Autodesk Fusion 360 part; units mm, degrees
(part 19 of 24)
  arc A6027 (67.5837, 18.8834) -> (67.2903, 18.7619) centre (67.437, 18.8226) ccw
  line L2242 (72.517, 13.6779) -> (72.517, 12.446)
  arc A6028 (74.5092, 15.1708) -> (74.6307, 14.8774) centre (74.57, 15.0241) ccw
  arc A6029 (72.6757, 12.446) -> (72.3582, 12.446) centre (72.517, 12.446) ccw
  line L2243 (78.673, 15.2859) -> (74.5249, 11.1379)
  arc A6030 (73.5901, 11.9357) -> (73.9076, 11.9357) centre (73.7489, 11.9357) ccw
  arc A6031 (75.5723, 15.8051) -> (75.5723, 15.4877) centre (75.5723, 15.6464) ccw
  arc A6032 (72.3583, 11.2141) -> (72.6758, 11.2141) centre (72.517, 11.2141) ccw
  arc A6033 (72.517, 11.3728) -> (72.517, 11.0554) centre (72.517, 11.2141) ccw
  line L2244 (74.5249, 11.1379) -> (72.1601, 11.1379)
  line L2245 (73.7489, 12.9563) -> (73.0273, 13.6779)
  line L2246 (75.2188, 15.2929) -> (75.5723, 15.6464)
  arc A6034 (72.517, 13.8366) -> (72.517, 13.5191) centre (72.517, 13.6779) ccw
  arc A6035 (73.7489, 12.2872) -> (73.7489, 12.6047) centre (73.7489, 12.446) ccw
  arc A6036 (72.517, 11.0553) -> (72.517, 11.3728) centre (72.517, 11.2141) ccw
  arc A6037 (73.9076, 12.9563) -> (73.5901, 12.9563) centre (73.7489, 12.9563) ccw
  line L2247 (72.517, 12.446) -> (72.517, 11.2141)
  arc A6038 (78.5607, 15.3982) -> (78.7852, 15.1737) centre (78.673, 15.286) ccw
  arc A6039 (72.1961, 11.3264) -> (71.9716, 11.1018) centre (72.0838, 11.2141) ccw
  line L2248 (73.0273, 13.6779) -> (72.517, 13.6779)
  arc A6040 (79.2149, 15.4997) -> (79.0934, 15.7931) centre (79.1542, 15.6464) ccw
  arc A6041 (73.8612, 11.8235) -> (73.6366, 12.048) centre (73.7489, 11.9358) ccw
  arc A6042 (72.1601, 11.2966) -> (72.1601, 10.9791) centre (72.1601, 11.1379) ccw
  line L2249 (75.5723, 15.6464) -> (79.1542, 15.6464)
  line L2250 (79.1542, 15.6464) -> (78.9481, 15.561)
  arc A6043 (75.1065, 15.4051) -> (75.331, 15.1806) centre (75.2188, 15.2929) ccw
  arc A6044 (79.1542, 15.4877) -> (79.1542, 15.8051) centre (79.1542, 15.6464) ccw
  line L2251 (78.9481, 15.561) -> (78.673, 15.2859)
  arc A6045 (74.5699, 14.8654) -> (74.5699, 15.1829) centre (74.5699, 15.0242) ccw
  arc A6046 (72.3583, 12.446) -> (72.6758, 12.446) centre (72.517, 12.446) ccw
  line L2252 (72.517, 11.2141) -> (73.0273, 11.2141)
  arc A6047 (73.1395, 13.7902) -> (72.915, 13.5656) centre (73.0272, 13.6779) ccw
  arc A6048 (74.5249, 10.9791) -> (74.5249, 11.2966) centre (74.5249, 11.1379) ccw
  arc A6049 (73.8677, 15.1829) -> (73.8677, 14.8654) centre (73.8677, 15.0242) ccw
  arc A6050 (73.9076, 12.446) -> (73.5901, 12.446) centre (73.7489, 12.446) ccw
  arc A6051 (78.8873, 15.7077) -> (79.0088, 15.4144) centre (78.948, 15.5611) ccw
  line L2253 (72.0839, 11.2141) -> (72.517, 11.2141)
  arc A6052 (72.0478, 11.0256) -> (72.2723, 11.2502) centre (72.16, 11.1379) ccw
  arc A6053 (72.517, 12.2872) -> (72.517, 12.6047) centre (72.517, 12.446) ccw
  arc A6054 (74.4127, 11.2502) -> (74.6372, 11.0256) centre (74.525, 11.1379) ccw
  arc A6055 (73.0273, 13.5191) -> (73.0273, 13.8366) centre (73.0273, 13.6779) ccw
  arc A6056 (72.6758, 12.446) -> (72.3583, 12.446) centre (72.517, 12.446) ccw
  arc A6057 (73.6366, 12.844) -> (73.8612, 13.0685) centre (73.7489, 12.9562) ccw
  arc A6058 (72.3582, 11.2141) -> (72.6757, 11.2141) centre (72.517, 11.2141) ccw
  arc A6059 (72.517, 12.6047) -> (72.517, 12.2872) centre (72.517, 12.446) ccw
  arc A6060 (72.3582, 12.446) -> (72.6757, 12.446) centre (72.517, 12.446) ccw
  arc A6061 (73.0273, 11.0554) -> (73.0273, 11.3728) centre (73.0273, 11.2141) ccw
  arc A6062 (78.7852, 15.1737) -> (78.5607, 15.3982) centre (78.673, 15.2859) ccw
  line L2254 (74.5699, 15.0241) -> (75.2188, 15.2929)
  arc A6063 (79.0603, 15.4488) -> (78.8358, 15.6733) centre (78.9481, 15.561) ccw
  line L2255 (73.7489, 11.9357) -> (73.7489, 12.446)
  line L2256 (72.517, 12.446) -> (73.7489, 12.446)
  arc A6064 (72.6757, 12.446) -> (72.3582, 12.446) centre (72.517, 12.446) ccw
  line L2257 (68.4989, 14.799) -> (68.1395, 14.9479)
  arc A6065 (71.1264, 12.0129) -> (71.4438, 12.0129) centre (71.2851, 12.0129) ccw
  arc A6066 (46.6957, 21.6967) -> (46.4024, 21.5752) centre (46.5491, 21.636) ccw
  line L2258 (72.517, 12.446) -> (72.517, 13.6779)
  arc A6067 (46.8566, 21.2765) -> (46.5391, 21.2765) centre (46.6979, 21.2765) ccw
  arc A6068 (72.517, 12.6048) -> (72.517, 12.2873) centre (72.517, 12.4461) ccw
  line L2259 (68.774, 14.5239) -> (68.4989, 14.799)
  arc A6069 (72.517, 12.6047) -> (72.517, 12.2872) centre (72.517, 12.446) ccw
  arc A6070 (68.6153, 14.5239) -> (68.9328, 14.5239) centre (68.7741, 14.5239) ccw
  arc A6071 (68.6618, 14.4117) -> (68.8863, 14.6362) centre (68.774, 14.524) ccw
  arc A6072 (72.915, 11.3264) -> (73.1395, 11.1018) centre (73.0272, 11.2141) ccw
  arc A6073 (46.8102, 18.2973) -> (46.5856, 18.0728) centre (46.6979, 18.185) ccw
  arc A6074 (46.5512, 21.2158) -> (46.8446, 21.3373) centre (46.6979, 21.2765) ccw
  line L2260 (46.6979, 21.2765) -> (46.549, 21.6359)
  line L2261 (72.0067, 13.6779) -> (71.2851, 12.9563)
  line L2262 (73.0273, 11.2141) -> (73.7489, 11.9357)
  arc A6075 (49.9351, 15.1066) -> (49.9351, 14.7891) centre (49.9351, 14.9479) ccw
  arc A6076 (68.8863, 14.6362) -> (68.6618, 14.4117) centre (68.7741, 14.5239) ccw
  arc A6077 (68.4382, 14.6524) -> (68.5597, 14.9457) centre (68.499, 14.7991) ccw
  line L2263 (49.9351, 14.9479) -> (46.6979, 18.1851)
  arc A6078 (72.3583, 12.446) -> (72.6758, 12.446) centre (72.517, 12.446) ccw
  arc A6079 (72.6757, 13.6779) -> (72.3582, 13.6779) centre (72.517, 13.6779) ccw
  arc A6080 (73.7489, 12.2873) -> (73.7489, 12.6048) centre (73.7489, 12.4461) ccw
  line L2264 (71.2851, 12.9563) -> (71.2851, 12.446)
  line L2265 (71.2851, 12.0129) -> (68.774, 14.5239)
  arc A6081 (72.6758, 12.446) -> (72.3583, 12.446) centre (72.517, 12.446) ccw
  line L2266 (73.7489, 12.446) -> (72.517, 12.446)
  line L2267 (72.1601, 11.1379) -> (72.0839, 11.2141)
  arc A6082 (72.0839, 11.3728) -> (72.0839, 11.0554) centre (72.0839, 11.2141) ccw
  arc A6083 (46.5391, 18.1851) -> (46.8566, 18.1851) centre (46.6979, 18.1851) ccw
  arc A6084 (72.517, 12.2873) -> (72.517, 12.6048) centre (72.517, 12.4461) ccw
  line L2268 (46.6979, 18.1851) -> (46.6979, 21.2765)
  arc A6085 (71.1728, 11.9006) -> (71.3974, 12.1251) centre (71.2851, 12.0129) ccw
  line L2269 (71.2851, 12.446) -> (71.2851, 12.0129)
  arc A6086 (72.3582, 12.446) -> (72.6757, 12.446) centre (72.517, 12.446) ccw
  arc A6087 (37.5797, 23.0188) -> (37.5797, 22.7012) centre (37.5797, 22.86) ccw
  arc A6088 (72.517, 13.5191) -> (72.517, 13.8366) centre (72.517, 13.6779) ccw
  arc A6089 (44.69, 23.6538) -> (44.69, 23.3362) centre (44.69, 23.495) ccw
  arc A6090 (36.0803, 22.7012) -> (36.0803, 23.0188) centre (36.0803, 22.86) ccw
  arc A6091 (29.21, 23.6538) -> (29.21, 23.3362) centre (29.21, 23.495) ccw
  arc A6092 (71.2851, 12.6047) -> (71.2851, 12.2872) centre (71.2851, 12.446) ccw
  arc A6093 (56.8579, 23.0188) -> (56.8579, 22.7012) centre (56.8579, 22.86) ccw
  line L2270 (71.2851, 12.446) -> (72.517, 12.446)
  arc A6094 (68.6112, 14.9113) -> (68.3867, 14.6868) centre (68.499, 14.799) ccw
  arc A6095 (72.517, 12.2872) -> (72.517, 12.6047) centre (72.517, 12.446) ccw
  arc A6096 (41.924, 23.3362) -> (41.924, 23.6538) centre (41.924, 23.495) ccw
  arc A6097 (49.8228, 14.8356) -> (50.0473, 15.0602) centre (49.9351, 14.9479) ccw
  arc A6098 (71.4438, 12.9563) -> (71.1264, 12.9563) centre (71.2851, 12.9563) ccw
  arc A6099 (32.4997, 23.0188) -> (32.4997, 22.7012) centre (32.4997, 22.86) ccw
  arc A6100 (47.5103, 22.7012) -> (47.5103, 23.0188) centre (47.5103, 22.86) ccw
  arc A6101 (68.2003, 15.0946) -> (68.0788, 14.8012) centre (68.1395, 14.9479) ccw
  arc A6102 (25.1591, 23.3362) -> (25.1591, 23.6538) centre (25.1591, 23.495) ccw
  arc A6103 (38.3409, 23.6538) -> (38.3409, 23.3362) centre (38.3409, 23.495) ccw
  arc A6104 (46.7491, 23.3362) -> (46.7491, 23.6538) centre (46.7491, 23.495) ccw
  line L2271 (72.517, 13.6779) -> (72.0067, 13.6779)
  arc A6105 (72.6758, 13.6779) -> (72.3583, 13.6779) centre (72.517, 13.6779) ccw
  arc A6106 (49.0097, 23.0188) -> (49.0097, 22.7012) centre (49.0097, 22.86) ccw
  line L2272 (72.517, 12.446) -> (71.2851, 12.446)
  arc A6107 (6.2857, 22.7012) -> (6.2857, 23.0188) centre (6.2857, 22.86) ccw
  arc A6108 (69.342, 22.7012) -> (69.342, 23.0188) centre (69.342, 22.86) ccw
  arc A6109 (68.1395, 14.7891) -> (68.1395, 15.1066) centre (68.1395, 14.9479) ccw
  arc A6110 (29.21, 23.3362) -> (29.21, 23.6538) centre (29.21, 23.495) ccw
  arc A6111 (72.0067, 13.8366) -> (72.0067, 13.5191) centre (72.0067, 13.6779) ccw
  arc A6112 (72.119, 13.5656) -> (71.8945, 13.7902) centre (72.0068, 13.6779) ccw
  arc A6113 (71.1264, 12.446) -> (71.4438, 12.446) centre (71.2851, 12.446) ccw
  arc A6114 (71.1728, 13.0685) -> (71.3974, 12.844) centre (71.2851, 12.9563) ccw
  arc A6115 (71.4438, 12.446) -> (71.1264, 12.446) centre (71.2851, 12.446) ccw
  arc A6116 (71.2851, 12.6048) -> (71.2851, 12.2873) centre (71.2851, 12.4461) ccw
  line L2273 (46.549, 21.6359) -> (46.2739, 21.911)
  line L2274 (12.3063, 33.5781) -> (12.5596, 32.9666)
  line L2275 (68.1395, 14.9479) -> (49.9351, 14.9479)
  arc A6117 (72.517, 12.2873) -> (72.517, 12.6048) centre (72.517, 12.4461) ccw
  arc A6118 (0.7747, 23.6538) -> (0.7747, 23.3362) centre (0.7747, 23.495) ccw
  arc A6119 (68.9328, 14.5239) -> (68.6153, 14.5239) centre (68.7741, 14.5239) ccw
  arc A6120 (7.62, 23.0188) -> (7.62, 22.7012) centre (7.62, 22.86) ccw
  arc A6121 (79.8488, 22.7012) -> (79.8488, 23.0188) centre (79.8488, 22.86) ccw
  arc A6122 (71.628, 24.2888) -> (71.628, 23.9713) centre (71.628, 24.1301) ccw
  arc A6123 (54.9021, 23.3362) -> (54.9021, 23.6538) centre (54.9021, 23.495) ccw
  arc A6124 (54.5068, 23.6538) -> (54.5068, 23.3362) centre (54.5068, 23.495) ccw
  arc A6125 (84.2253, 22.7012) -> (84.2253, 23.0188) centre (84.2253, 22.86) ccw
  arc A6126 (53.34, 23.3362) -> (53.34, 23.6538) centre (53.34, 23.495) ccw
  arc A6127 (71.628, 23.0188) -> (71.628, 22.7012) centre (71.628, 22.86) ccw
  arc A6128 (45.325, 23.0188) -> (45.325, 22.7012) centre (45.325, 22.86) ccw
  arc A6129 (25.9203, 22.7012) -> (25.9203, 23.0188) centre (25.9203, 22.86) ccw
  arc A6130 (33.5403, 22.7012) -> (33.5403, 23.0188) centre (33.5403, 22.86) ccw
  arc A6131 (42.559, 22.7012) -> (42.559, 23.0188) centre (42.559, 22.86) ccw
  arc A6132 (75.0912, 23.0188) -> (75.0912, 22.7012) centre (75.0912, 22.86) ccw
  arc A6133 (73.3464, 22.7012) -> (73.3464, 23.0188) centre (73.3464, 22.86) ccw
  arc A6134 (83.5279, 23.0188) -> (83.5279, 22.7012) centre (83.5279, 22.86) ccw
  arc A6135 (83.298, 22.3838) -> (83.298, 22.0663) centre (83.298, 22.2251) ccw
  arc A6136 (53.34, 23.6538) -> (53.34, 23.3362) centre (53.34, 23.495) ccw
  arc A6137 (0.7747, 23.0188) -> (0.7747, 22.7012) centre (0.7747, 22.86) ccw
  arc A6138 (27.4197, 23.0188) -> (27.4197, 22.7012) centre (27.4197, 22.86) ccw
  arc A6139 (54.9021, 22.7012) -> (54.9021, 23.0188) centre (54.9021, 22.86) ccw
  arc A6140 (7.62, 22.7012) -> (7.62, 23.0188) centre (7.62, 22.86) ccw
  arc A6141 (71.628, 22.3838) -> (71.628, 22.0663) centre (71.628, 22.2251) ccw
  arc A6142 (8.9543, 23.0188) -> (8.9543, 22.7012) centre (8.9543, 22.86) ccw
  arc A6143 (31.0003, 22.7012) -> (31.0003, 23.0188) centre (31.0003, 22.86) ccw
  arc A6144 (35.0397, 23.0188) -> (35.0397, 22.7012) centre (35.0397, 22.86) ccw
  arc A6145 (51.5497, 23.0188) -> (51.5497, 22.7012) centre (51.5497, 22.86) ccw
  arc A6146 (50.0503, 22.7012) -> (50.0503, 23.0188) centre (50.0503, 22.86) ccw
  arc A6147 (84.2253, 22.0663) -> (84.2253, 22.3838) centre (84.2253, 22.2251) ccw
  arc A6148 (44.972, 24.6062) -> (44.972, 24.9238) centre (44.972, 24.765) ccw
  arc A6149 (81.5721, 23.3362) -> (81.5721, 23.6538) centre (81.5721, 23.495) ccw
  arc A6150 (46.4947, 23.9713) -> (46.4947, 24.2888) centre (46.4947, 24.1301) ccw
  arc A6151 (29.21, 24.9238) -> (29.21, 24.6062) centre (29.21, 24.765) ccw
  arc A6152 (54.9021, 24.6062) -> (54.9021, 24.9238) centre (54.9021, 24.765) ccw
  arc A6153 (59.8864, 24.9238) -> (59.8864, 24.6062) centre (59.8864, 24.765) ccw
  arc A6154 (72.39, 24.6062) -> (72.39, 24.9238) centre (72.39, 24.765) ccw
  arc A6155 (56.8579, 23.6538) -> (56.8579, 23.3362) centre (56.8579, 23.495) ccw
  arc A6156 (24.9047, 23.9713) -> (24.9047, 24.2888) centre (24.9047, 24.1301) ccw
  arc A6157 (56.9536, 24.6062) -> (56.9536, 24.9238) centre (56.9536, 24.765) ccw
  arc A6158 (84.2253, 23.9713) -> (84.2253, 24.2888) centre (84.2253, 24.1301) ccw
  arc A6159 (40.816, 24.6062) -> (40.816, 24.9238) centre (40.816, 24.765) ccw
  arc A6160 (68.58, 24.6062) -> (68.58, 24.9238) centre (68.58, 24.765) ccw
  arc A6161 (53.34, 24.2888) -> (53.34, 23.9713) centre (53.34, 24.1301) ccw
  arc A6162 (44.055, 24.2888) -> (44.055, 23.9713) centre (44.055, 24.1301) ccw
  arc A6163 (43.42, 24.9238) -> (43.42, 24.6062) centre (43.42, 24.765) ccw
  arc A6164 (53.34, 24.9238) -> (53.34, 24.6062) centre (53.34, 24.765) ccw
  arc A6165 (69.342, 23.9713) -> (69.342, 24.2888) centre (69.342, 24.1301) ccw
  arc A6166 (41.289, 23.9713) -> (41.289, 24.2888) centre (41.289, 24.1301) ccw
  arc A6167 (57.5886, 23.9713) -> (57.5886, 24.2888) centre (57.5886, 24.1301) ccw
  arc A6168 (54.9021, 23.9713) -> (54.9021, 24.2888) centre (54.9021, 24.1301) ccw
  arc A6169 (38.5953, 24.9238) -> (38.5953, 24.6062) centre (38.5953, 24.765) ccw
  arc A6170 (54.8513, 24.9238) -> (54.8513, 24.6062) centre (54.8513, 24.765) ccw
  arc A6171 (72.39, 24.9238) -> (72.39, 24.6062) centre (72.39, 24.765) ccw
  arc A6172 (53.34, 24.6062) -> (53.34, 24.9238) centre (53.34, 24.765) ccw
  arc A6173 (67.4728, 24.6062) -> (67.4728, 24.9238) centre (67.4728, 24.765) ccw
  arc A6174 (68.58, 24.9238) -> (68.58, 24.6062) centre (68.58, 24.765) ccw
  arc A6175 (54.8178, 24.2888) -> (54.8178, 23.9713) centre (54.8178, 24.1301) ccw
  arc A6176 (71.628, 23.6538) -> (71.628, 23.3362) centre (71.628, 23.495) ccw
  arc A6177 (0.7747, 24.2888) -> (0.7747, 23.9713) centre (0.7747, 24.1301) ccw
  arc A6178 (83.5279, 24.2888) -> (83.5279, 23.9713) centre (83.5279, 24.1301) ccw
  arc A6179 (54.9021, 25.2413) -> (54.9021, 25.5588) centre (54.9021, 25.4001) ccw
  arc A6180 (59.2514, 24.2888) -> (59.2514, 23.9713) centre (59.2514, 24.1301) ccw
  arc A6181 (83.5279, 23.6538) -> (83.5279, 23.3362) centre (83.5279, 23.495) ccw
  arc A6182 (43.1637, 25.5588) -> (43.1637, 25.2413) centre (43.1637, 25.4001) ccw
  arc A6183 (0.7747, 24.9238) -> (0.7747, 24.6062) centre (0.7747, 24.765) ccw
  arc A6184 (81.5721, 23.9713) -> (81.5721, 24.2888) centre (81.5721, 24.1301) ccw
  arc A6185 (56.8579, 24.2888) -> (56.8579, 23.9713) centre (56.8579, 24.1301) ccw
  arc A6186 (84.0359, 25.5588) -> (84.0359, 25.2413) centre (84.0359, 25.4001) ccw
  arc A6187 (59.8864, 26.1938) -> (59.8864, 25.8762) centre (59.8864, 26.035) ccw
  arc A6188 (29.21, 24.2888) -> (29.21, 23.9713) centre (29.21, 24.1301) ccw
  arc A6189 (84.2253, 23.3362) -> (84.2253, 23.6538) centre (84.2253, 23.495) ccw
  arc A6190 (56.8579, 24.9238) -> (56.8579, 24.6062) centre (56.8579, 24.765) ccw
  arc A6191 (68.58, 25.8762) -> (68.58, 26.1938) centre (68.58, 26.035) ccw
  arc A6192 (15.4854, 24.6062) -> (15.4854, 24.9238) centre (15.4854, 24.765) ccw
  arc A6193 (73.4972, 26.1938) -> (73.4972, 25.8762) centre (73.4972, 26.035) ccw
  arc A6194 (14.7483, 25.8762) -> (14.7483, 26.1938) centre (14.7483, 26.035) ccw
  arc A6195 (68.58, 25.2413) -> (68.58, 25.5588) centre (68.58, 25.4001) ccw
  arc A6196 (84.0164, 26.1938) -> (84.0164, 25.8762) centre (84.0164, 26.035) ccw
  arc A6197 (69.342, 23.3362) -> (69.342, 23.6538) centre (69.342, 23.495) ccw
  arc A6198 (53.34, 23.9713) -> (53.34, 24.2888) centre (53.34, 24.1301) ccw
  arc A6199 (38.5953, 25.5588) -> (38.5953, 25.2413) centre (38.5953, 25.4001) ccw
  arc A6200 (59.9059, 25.5588) -> (59.9059, 25.2413) centre (59.9059, 25.4001) ccw
  arc A6201 (38.5953, 24.2888) -> (38.5953, 23.9713) centre (38.5953, 24.1301) ccw
  arc A6202 (29.21, 24.6062) -> (29.21, 24.9238) centre (29.21, 24.765) ccw
  arc A6203 (43.702, 25.8762) -> (43.702, 26.1938) centre (43.702, 26.035) ccw
  arc A6204 (53.34, 25.8762) -> (53.34, 26.1938) centre (53.34, 26.035) ccw
  arc A6205 (81.0836, 24.6062) -> (81.0836, 24.9238) centre (81.0836, 24.765) ccw
  arc A6206 (53.34, 25.5588) -> (53.34, 25.2413) centre (53.34, 25.4001) ccw
  arc A6207 (14.8554, 25.2413) -> (14.8554, 25.5588) centre (14.8554, 25.4001) ccw
  arc A6208 (72.39, 26.1938) -> (72.39, 25.8762) centre (72.39, 26.035) ccw
  arc A6209 (14.991, 26.5113) -> (14.991, 26.8288) centre (14.991, 26.67) ccw
  arc A6210 (72.39, 25.8762) -> (72.39, 26.1938) centre (72.39, 26.035) ccw
  arc A6211 (29.21, 23.9713) -> (29.21, 24.2888) centre (29.21, 24.1301) ccw
  arc A6212 (40.6563, 25.2413) -> (40.6563, 25.5588) centre (40.6563, 25.4001) ccw
  arc A6213 (54.8513, 26.1938) -> (54.8513, 25.8762) centre (54.8513, 26.035) ccw
  arc A6214 (0.7747, 25.5588) -> (0.7747, 25.2413) centre (0.7747, 25.4001) ccw
  arc A6215 (84.2253, 25.8762) -> (84.2253, 26.1938) centre (84.2253, 26.035) ccw
  arc A6216 (53.34, 26.1938) -> (53.34, 25.8762) centre (53.34, 26.035) ccw
  arc A6217 (68.58, 26.1938) -> (68.58, 25.8762) centre (68.58, 26.035) ccw
  arc A6218 (29.21, 26.1938) -> (29.21, 25.8762) centre (29.21, 26.035) ccw
  arc A6219 (0.7747, 26.1938) -> (0.7747, 25.8762) centre (0.7747, 26.035) ccw
  arc A6220 (44.337, 25.2413) -> (44.337, 25.5588) centre (44.337, 25.4001) ccw
  arc A6221 (56.9536, 25.8762) -> (56.9536, 26.1938) centre (56.9536, 26.035) ccw
  arc A6222 (0.7747, 26.8288) -> (0.7747, 26.5113) centre (0.7747, 26.67) ccw
  arc A6223 (37.5797, 28.0988) -> (37.5797, 27.7813) centre (37.5797, 27.9401) ccw
  arc A6224 (54.9021, 27.7813) -> (54.9021, 28.0988) centre (54.9021, 27.9401) ccw
  arc A6225 (51.943, 28.0988) -> (51.943, 27.7813) centre (51.943, 27.9401) ccw
  arc A6226 (84.2253, 26.5113) -> (84.2253, 26.8288) centre (84.2253, 26.67) ccw
  arc A6227 (83.3814, 26.8288) -> (83.3814, 26.5113) centre (83.3814, 26.67) ccw
  arc A6228 (84.0164, 24.9238) -> (84.0164, 24.6062) centre (84.0164, 24.765) ccw
  arc A6229 (56.8579, 26.1938) -> (56.8579, 25.8762) centre (56.8579, 26.035) ccw
  arc A6230 (40.816, 25.8762) -> (40.816, 26.1938) centre (40.816, 26.035) ccw
  arc A6231 (43.004, 26.1938) -> (43.004, 25.8762) centre (43.004, 26.035) ccw
  arc A6232 (73.4972, 24.9238) -> (73.4972, 24.6062) centre (73.4972, 24.765) ccw
  arc A6233 (56.8579, 25.5588) -> (56.8579, 25.2413) centre (56.8579, 25.4001) ccw
  arc A6234 (38.5953, 26.1938) -> (38.5953, 25.8762) centre (38.5953, 26.035) ccw
  arc A6235 (81.0836, 25.8762) -> (81.0836, 26.1938) centre (81.0836, 26.035) ccw
  arc A6236 (84.2253, 25.2413) -> (84.2253, 25.5588) centre (84.2253, 25.4001) ccw
  arc A6237 (84.2253, 24.6062) -> (84.2253, 24.9238) centre (84.2253, 24.765) ccw
  arc A6238 (54.9021, 25.8762) -> (54.9021, 26.1938) centre (54.9021, 26.035) ccw
  arc A6239 (81.0641, 25.2413) -> (81.0641, 25.5588) centre (81.0641, 25.4001) ccw
  arc A6240 (29.21, 25.8762) -> (29.21, 26.1938) centre (29.21, 26.035) ccw
  arc A6241 (72.39, 25.5588) -> (72.39, 25.2413) centre (72.39, 25.4001) ccw
  arc A6242 (56.9341, 25.2413) -> (56.9341, 25.5588) centre (56.9341, 25.4001) ccw
  arc A6243 (67.4728, 25.8762) -> (67.4728, 26.1938) centre (67.4728, 26.035) ccw
  arc A6244 (29.21, 27.1462) -> (29.21, 27.4638) centre (29.21, 27.305) ccw
  arc A6245 (84.2253, 27.7813) -> (84.2253, 28.0988) centre (84.2253, 27.9401) ccw
  arc A6246 (43.067, 26.5113) -> (43.067, 26.8288) centre (43.067, 26.67) ccw
  arc A6247 (36.0803, 27.7813) -> (36.0803, 28.0988) centre (36.0803, 27.9401) ccw
  arc A6248 (81.7186, 26.5113) -> (81.7186, 26.8288) centre (81.7186, 26.67) ccw
  arc A6249 (53.34, 27.4638) -> (53.34, 27.1462) centre (53.34, 27.305) ccw
  arc A6250 (41.797, 27.7813) -> (41.797, 28.0988) centre (41.797, 27.9401) ccw
  arc A6251 (73.3714, 27.4638) -> (73.3714, 27.1462) centre (73.3714, 27.305) ccw
  arc A6252 (38.5953, 26.8288) -> (38.5953, 26.5113) centre (38.5953, 26.67) ccw
  arc A6253 (63.1536, 27.7813) -> (63.1536, 28.0988) centre (63.1536, 27.9401) ccw
  arc A6254 (27.813, 28.0988) -> (27.813, 27.7813) centre (27.813, 27.9401) ccw
  arc A6255 (42.432, 27.1462) -> (42.432, 27.4638) centre (42.432, 27.305) ccw
  arc A6256 (84.2253, 27.1462) -> (84.2253, 27.4638) centre (84.2253, 27.305) ccw
  arc A6257 (54.9021, 26.5113) -> (54.9021, 26.8288) centre (54.9021, 26.67) ccw
  arc A6258 (57.5886, 26.5113) -> (57.5886, 26.8288) centre (57.5886, 26.67) ccw
  arc A6259 (56.8579, 28.0988) -> (56.8579, 27.7813) centre (56.8579, 27.9401) ccw
  arc A6260 (29.21, 26.5113) -> (29.21, 26.8288) centre (29.21, 26.67) ccw
  arc A6261 (53.34, 26.5113) -> (53.34, 26.8288) centre (53.34, 26.67) ccw
  arc A6262 (5.9265, 27.7813) -> (5.9265, 28.0988) centre (5.9265, 27.9401) ccw
  arc A6263 (69.342, 26.5113) -> (69.342, 26.8288) centre (69.342, 26.67) ccw
  arc A6264 (33.5403, 27.7813) -> (33.5403, 28.0988) centre (33.5403, 27.9401) ccw
  arc A6265 (29.21, 26.8288) -> (29.21, 26.5113) centre (29.21, 26.67) ccw
sketch "Top Component Outlines" plane through (0, 0, 0) normal (0, 0, 1) x (1, 0, 0)
  arc A0 (71.501, 48.2981) -> (71.501, 48.2219) centre (71.501, 48.26) ccw
  arc A1 (71.501, 48.2219) -> (71.501, 48.2981) centre (71.501, 48.26) ccw
  arc A2 (76.0349, 48.514) -> (76.1111, 48.514) centre (76.073, 48.514) ccw
  arc A3 (73.9775, 50.292) -> (73.8505, 50.292) centre (73.914, 50.292) ccw
  arc A4 (75.819, 48.2219) -> (75.819, 48.2981) centre (75.819, 48.26) ccw
  arc A5 (73.9775, 49.53) -> (73.8505, 49.53) centre (73.914, 49.53) ccw
  arc A6 (71.501, 50.8) -> (71.247, 50.546) centre (71.501, 50.546) ccw
  arc A7 (76.1111, 50.546) -> (76.0349, 50.546) centre (76.073, 50.546) ccw
  arc A8 (71.501, 50.7619) -> (71.501, 50.8381) centre (71.501, 50.8) ccw
  arc A9 (73.3425, 49.53) -> (73.4695, 49.53) centre (73.406, 49.53) ccw
  arc A10 (71.501, 50.8381) -> (71.501, 50.7619) centre (71.501, 50.8) ccw
  arc A11 (71.2851, 48.514) -> (71.2089, 48.514) centre (71.247, 48.514) ccw
  arc A12 (73.3425, 48.768) -> (73.4695, 48.768) centre (73.406, 48.768) ccw
  line L0 (74.041, 49.53) -> (73.914, 49.53)
  line L1 (71.247, 50.546) -> (71.247, 48.514)
  arc A13 (71.2089, 48.514) -> (71.2851, 48.514) centre (71.247, 48.514) ccw
  line L2 (71.501, 50.8) -> (75.819, 50.8)
  arc A14 (76.0349, 50.546) -> (76.1111, 50.546) centre (76.073, 50.546) ccw
  arc A15 (76.1111, 48.514) -> (76.0349, 48.514) centre (76.073, 48.514) ccw
  arc A16 (71.2089, 50.546) -> (71.2851, 50.546) centre (71.247, 50.546) ccw
  line L3 (73.914, 49.53) -> (73.914, 48.768)
  line L4 (75.819, 48.26) -> (71.501, 48.26)
  arc A17 (71.247, 48.514) -> (71.501, 48.26) centre (71.501, 48.514) ccw
  arc A18 (73.4695, 50.292) -> (73.3425, 50.292) centre (73.406, 50.292) ccw
  arc A19 (75.819, 50.8381) -> (75.819, 50.7619) centre (75.819, 50.8) ccw
  arc A20 (73.914, 49.5681) -> (73.914, 49.4919) centre (73.914, 49.53) ccw
  arc A21 (74.041, 49.4919) -> (74.041, 49.5681) centre (74.041, 49.53) ccw
  arc A22 (76.073, 50.546) -> (75.819, 50.8) centre (75.819, 50.546) ccw
  arc A23 (75.819, 50.7619) -> (75.819, 50.8381) centre (75.819, 50.8) ccw
  arc A24 (71.2851, 50.546) -> (71.2089, 50.546) centre (71.247, 50.546) ccw
  arc A25 (75.819, 48.26) -> (76.073, 48.514) centre (75.819, 48.514) ccw
  arc A26 (75.819, 48.2981) -> (75.819, 48.2219) centre (75.819, 48.26) ccw
  line L5 (73.406, 49.53) -> (73.279, 49.53)
  arc A27 (73.406, 49.4919) -> (73.406, 49.5681) centre (73.406, 49.53) ccw
  arc A28 (73.8505, 49.53) -> (73.9775, 49.53) centre (73.914, 49.53) ccw
  arc A29 (73.4695, 49.53) -> (73.3425, 49.53) centre (73.406, 49.53) ccw
  arc A30 (73.279, 49.5681) -> (73.279, 49.4919) centre (73.279, 49.53) ccw
  line L6 (76.073, 50.546) -> (76.073, 48.514)
  arc A31 (73.8505, 48.768) -> (73.9775, 48.768) centre (73.914, 48.768) ccw
  line L7 (73.914, 49.53) -> (73.914, 50.292)
  line L8 (73.406, 50.292) -> (73.406, 49.53)
  line L9 (73.406, 49.53) -> (73.406, 48.768)
  arc A32 (14.605, 38.9509) -> (14.605, 39.0271) centre (14.605, 38.989) ccw
  line L10 (12.7, 37.338) -> (15.24, 37.338)
  line L11 (15.24, 37.338) -> (15.24, 37.846)
  line L12 (13.97, 38.989) -> (14.605, 38.989)
  arc A33 (13.97, 39.0271) -> (13.97, 38.9509) centre (13.97, 38.989) ccw
  arc A34 (15.2019, 36.957) -> (15.2781, 36.957) centre (15.24, 36.957) ccw
  arc A35 (50.3809, 18.669) -> (50.4571, 18.669) centre (50.419, 18.669) ccw
  line L13 (13.97, 38.354) -> (13.97, 38.989)
  arc A36 (14.605, 39.9669) -> (14.605, 40.0431) centre (14.605, 40.005) ccw
  line L14 (14.351, 41.021) -> (14.351, 42.926)
  arc A37 (50.4571, 19.05) -> (50.3809, 19.05) centre (50.419, 19.05) ccw
  arc A38 (52.07, 20.574) -> (52.07, 14.986) centre (52.07, 17.78) ccw
  arc A39 (15.2781, 41.021) -> (15.2019, 41.021) centre (15.24, 41.021) ccw
  line L15 (13.589, 36.957) -> (13.589, 35.052)
  arc A40 (15.24, 36.9189) -> (15.24, 36.9951) centre (15.24, 36.957) ccw
  line L16 (13.589, 35.052) -> (14.351, 35.052)
  arc A41 (52.07, 14.986) -> (52.07, 20.574) centre (52.07, 17.78) ccw
  line L17 (14.351, 42.926) -> (13.589, 42.926)
  line L18 (50.419, 19.05) -> (50.419, 19.431)
  line L19 (13.335, 40.005) -> (14.605, 40.005)
  arc A42 (13.9319, 38.354) -> (14.0081, 38.354) centre (13.97, 38.354) ccw
  line L20 (15.24, 37.846) -> (12.7, 37.846)
  arc A43 (14.0081, 38.989) -> (13.9319, 38.989) centre (13.97, 38.989) ccw
  line L21 (13.335, 38.989) -> (13.97, 38.989)
  arc A44 (12.7, 41.0591) -> (12.7, 40.9829) centre (12.7, 41.021) ccw
  line L22 (13.589, 41.021) -> (14.351, 41.021)
  line L23 (14.605, 40.005) -> (13.97, 38.989)
  arc A45 (50.4571, 19.431) -> (50.3809, 19.431) centre (50.419, 19.431) ccw
  arc A46 (50.038, 19.0881) -> (50.038, 19.0119) centre (50.038, 19.05) ccw
  line L24 (13.97, 38.989) -> (13.335, 40.005)
  arc A47 (15.24, 40.9829) -> (15.24, 41.0591) centre (15.24, 41.021) ccw
  line L25 (15.24, 41.021) -> (15.24, 36.957)
  line L26 (50.419, 18.669) -> (50.419, 19.05)
  arc A48 (12.7381, 41.021) -> (12.6619, 41.021) centre (12.7, 41.021) ccw
  arc A49 (13.9377, 39.0092) -> (14.0023, 38.9688) centre (13.97, 38.989) ccw
  arc A50 (12.7, 36.9951) -> (12.7, 36.9189) centre (12.7, 36.957) ccw
  arc A51 (14.0081, 40.513) -> (13.9319, 40.513) centre (13.97, 40.513) ccw
  arc A52 (13.3673, 40.0252) -> (13.3027, 39.9848) centre (13.335, 40.005) ccw
  arc A53 (13.9377, 38.9688) -> (14.0023, 39.0092) centre (13.97, 38.989) ccw
  arc A54 (13.335, 39.0271) -> (13.335, 38.9509) centre (13.335, 38.989) ccw
  line L27 (13.589, 42.926) -> (13.589, 41.021)
  line L28 (13.97, 38.989) -> (13.97, 40.513)
  arc A55 (13.97, 38.9509) -> (13.97, 39.0271) centre (13.97, 38.989) ccw
  line L29 (12.7, 37.846) -> (12.7, 37.338)
  arc A56 (50.419, 19.0119) -> (50.419, 19.0881) centre (50.419, 19.05) ccw
  line L30 (12.7, 36.957) -> (12.7, 41.021)
  arc A57 (13.9319, 38.989) -> (14.0081, 38.989) centre (13.97, 38.989) ccw
  arc A58 (14.6373, 39.9848) -> (14.5727, 40.0252) centre (14.605, 40.005) ccw
  arc A59 (13.335, 40.0431) -> (13.335, 39.9669) centre (13.335, 40.005) ccw
  arc A60 (25.3492, 24.765) -> (25.4508, 24.765) centre (25.4, 24.765) ccw
  arc A61 (50.8, 19.0119) -> (50.8, 19.0881) centre (50.8, 19.05) ccw
  line L31 (12.7, 36.957) -> (15.24, 36.957)
  line L32 (25.4, 26.035) -> (25.4, 24.765)
  arc A62 (50.3809, 19.05) -> (50.4571, 19.05) centre (50.419, 19.05) ccw
  arc A63 (12.6619, 36.957) -> (12.7381, 36.957) centre (12.7, 36.957) ccw
  arc A64 (50.419, 19.0881) -> (50.419, 19.0119) centre (50.419, 19.05) ccw
  line L33 (14.351, 36.957) -> (13.589, 36.957)
  line L34 (15.24, 41.021) -> (12.7, 41.021)
  line L35 (14.351, 35.052) -> (14.351, 36.957)
  line L36 (50.038, 19.05) -> (50.419, 19.05)
  line L37 (50.419, 19.05) -> (50.8, 19.05)
  line L38 (72.39, 45.085) -> (72.39, 43.815)
  arc A65 (72.3392, 43.815) -> (72.4408, 43.815) centre (72.39, 43.815) ccw
  arc A66 (25.4508, 26.035) -> (25.3492, 26.035) centre (25.4, 26.035) ccw
  arc A67 (72.4408, 45.085) -> (72.3392, 45.085) centre (72.39, 45.085) ccw
  line L39 (38.1, 26.035) -> (38.1, 24.765)
  arc A68 (82.6008, 32.385) -> (82.4992, 32.385) centre (82.55, 32.385) ccw
  line L40 (82.55, 32.385) -> (82.55, 31.115)
  arc A69 (82.4992, 31.115) -> (82.6008, 31.115) centre (82.55, 31.115) ccw
  arc A70 (38.1508, 26.035) -> (38.0492, 26.035) centre (38.1, 26.035) ccw
  arc A71 (67.3608, 43.815) -> (67.2592, 43.815) centre (67.31, 43.815) ccw
  line L41 (57.15, 43.815) -> (57.15, 42.545)
  line L42 (59.69, 31.115) -> (59.69, 32.385)
  arc A72 (22.9108, 50.165) -> (22.8092, 50.165) centre (22.86, 50.165) ccw
  arc A73 (22.8092, 48.895) -> (22.9108, 48.895) centre (22.86, 48.895) ccw
  arc A74 (57.2008, 43.815) -> (57.0992, 43.815) centre (57.15, 43.815) ccw
  arc A75 (33.0962, 37.9476) -> (33.0962, 38.2524) centre (33.0962, 38.1) ccw
  arc A76 (72.4408, 32.385) -> (72.3392, 32.385) centre (72.39, 32.385) ccw
  arc A77 (59.7408, 32.385) -> (59.6392, 32.385) centre (59.69, 32.385) ccw
  arc A78 (67.2592, 42.545) -> (67.3608, 42.545) centre (67.31, 42.545) ccw
  arc A79 (27.8638, 38.2524) -> (27.8638, 37.9476) centre (27.8638, 38.1) ccw
  line L43 (33.0962, 38.1) -> (27.8638, 38.1)
  arc A80 (72.3392, 31.115) -> (72.4408, 31.115) centre (72.39, 31.115) ccw
  arc A81 (67.3608, 32.385) -> (67.2592, 32.385) centre (67.31, 32.385) ccw
  arc A82 (67.2592, 31.115) -> (67.3608, 31.115) centre (67.31, 31.115) ccw
  arc A83 (59.6392, 31.115) -> (59.7408, 31.115) centre (59.69, 31.115) ccw
  line L44 (22.86, 48.895) -> (22.86, 50.165)
  arc A84 (33.0962, 34.1376) -> (33.0962, 34.4424) centre (33.0962, 34.29) ccw
  line L45 (72.39, 32.385) -> (72.39, 31.115)
  arc A85 (57.0992, 42.545) -> (57.2008, 42.545) centre (57.15, 42.545) ccw
  line L46 (33.0962, 34.29) -> (27.8638, 34.29)
  arc A86 (46.9392, 24.765) -> (47.0408, 24.765) centre (46.99, 24.765) ccw
  line L47 (54.61, 26.035) -> (54.61, 24.765)
  arc A87 (54.5592, 24.765) -> (54.6608, 24.765) centre (54.61, 24.765) ccw
  arc A88 (82.4992, 43.815) -> (82.6008, 43.815) centre (82.55, 43.815) ccw
  arc A89 (38.0492, 24.765) -> (38.1508, 24.765) centre (38.1, 24.765) ccw
  arc A90 (82.6008, 45.085) -> (82.4992, 45.085) centre (82.55, 45.085) ccw
  arc A91 (10.1092, 48.895) -> (10.2108, 48.895) centre (10.16, 48.895) ccw
  arc A92 (27.8638, 34.4424) -> (27.8638, 34.1376) centre (27.8638, 34.29) ccw
  line L48 (82.55, 45.085) -> (82.55, 43.815)
  line L49 (10.16, 48.895) -> (10.16, 50.165)
  line L50 (67.31, 31.115) -> (67.31, 32.385)
  arc A93 (10.2108, 50.165) -> (10.1092, 50.165) centre (10.16, 50.165) ccw
  line L51 (67.31, 43.815) -> (67.31, 42.545)
  line L52 (34.925, 15.24) -> (34.29, 15.875)
  arc A94 (36.8659, 15.8391) -> (36.7941, 15.9109) centre (36.83, 15.875) ccw
  arc A95 (34.2541, 17.1809) -> (34.3259, 17.1091) centre (34.29, 17.145) ccw
  arc A96 (38.6991, 15.2759) -> (38.7709, 15.2041) centre (38.735, 15.24) ccw
  arc A97 (39.4059, 15.8391) -> (39.3341, 15.9109) centre (39.37, 15.875) ccw
  line L53 (36.195, 15.24) -> (34.925, 15.24)
  line L54 (29.845, 17.78) -> (31.115, 17.78)
  arc A98 (29.8809, 17.7441) -> (29.8091, 17.8159) centre (29.845, 17.78) ccw
  line L55 (26.67, 17.145) -> (27.305, 17.78)
  line L56 (46.99, 26.035) -> (46.99, 24.765)
  line L57 (37.465, 17.78) -> (36.83, 17.145)
  arc A99 (31.0791, 15.2759) -> (31.1509, 15.2041) centre (31.115, 15.24) ccw
  arc A100 (37.5009, 17.7441) -> (37.4291, 17.8159) centre (37.465, 17.78) ccw
  line L58 (34.925, 17.78) -> (36.195, 17.78)
  line L59 (31.115, 17.78) -> (31.75, 17.145)
  arc A101 (31.1509, 17.8159) -> (31.0791, 17.7441) centre (31.115, 17.78) ccw
  arc A102 (39.3341, 17.1091) -> (39.4059, 17.1809) centre (39.37, 17.145) ccw
  line L60 (36.83, 15.875) -> (36.195, 15.24)
  arc A103 (36.2309, 17.8159) -> (36.1591, 17.7441) centre (36.195, 17.78) ccw
  arc A104 (36.7941, 17.1091) -> (36.8659, 17.1809) centre (36.83, 17.145) ccw
  arc A105 (34.925, 15.2908) -> (34.925, 15.1892) centre (34.925, 15.24) ccw
  arc A106 (36.195, 15.1892) -> (36.195, 15.2908) centre (36.195, 15.24) ccw
  arc A107 (36.7941, 17.1809) -> (36.8659, 17.1091) centre (36.83, 17.145) ccw
  arc A108 (37.465, 17.8308) -> (37.465, 17.7292) centre (37.465, 17.78) ccw
  arc A109 (38.735, 17.7292) -> (38.735, 17.8308) centre (38.735, 17.78) ccw
  line L61 (37.465, 17.78) -> (38.735, 17.78)
  arc A110 (38.7709, 17.8159) -> (38.6991, 17.7441) centre (38.735, 17.78) ccw
  arc A111 (36.195, 17.7292) -> (36.195, 17.8308) centre (36.195, 17.78) ccw
  line L62 (36.195, 17.78) -> (36.83, 17.145)
  arc A112 (34.8891, 15.2041) -> (34.9609, 15.2759) centre (34.925, 15.24) ccw
  arc A113 (34.925, 17.8308) -> (34.925, 17.7292) centre (34.925, 17.78) ccw
  line L63 (36.83, 15.875) -> (37.465, 15.24)
  arc A114 (31.115, 17.7292) -> (31.115, 17.8308) centre (31.115, 17.78) ccw
  arc A115 (54.6608, 26.035) -> (54.5592, 26.035) centre (54.61, 26.035) ccw
  arc A116 (47.0408, 26.035) -> (46.9392, 26.035) centre (46.99, 26.035) ccw
  line L64 (34.29, 17.145) -> (34.925, 17.78)
  arc A117 (36.1591, 15.2759) -> (36.2309, 15.2041) centre (36.195, 15.24) ccw
  arc A118 (34.3259, 15.9109) -> (34.2541, 15.8391) centre (34.29, 15.875) ccw
  arc A119 (38.735, 15.1892) -> (38.735, 15.2908) centre (38.735, 15.24) ccw
  arc A120 (34.9609, 17.7441) -> (34.8891, 17.8159) centre (34.925, 17.78) ccw
  arc A121 (29.845, 17.8308) -> (29.845, 17.7292) centre (29.845, 17.78) ccw
  arc A122 (37.4291, 15.2041) -> (37.5009, 15.2759) centre (37.465, 15.24) ccw
  arc A123 (36.8659, 15.9109) -> (36.7941, 15.8391) centre (36.83, 15.875) ccw
  line L65 (31.75, 15.875) -> (31.115, 15.24)
  line L66 (38.735, 17.78) -> (39.37, 17.145)
  arc A124 (37.465, 15.2908) -> (37.465, 15.1892) centre (37.465, 15.24) ccw
  arc A125 (31.7141, 17.1091) -> (31.7859, 17.1809) centre (31.75, 17.145) ccw
  line L67 (38.735, 15.24) -> (37.465, 15.24)
  line L68 (39.37, 15.875) -> (38.735, 15.24)
  line L69 (31.75, 17.145) -> (32.385, 17.78)
  arc A126 (27.2691, 15.2041) -> (27.3409, 15.2759) centre (27.305, 15.24) ccw
  arc A127 (29.845, 15.2908) -> (29.845, 15.1892) centre (29.845, 15.24) ccw
  line L70 (24.13, 17.145) -> (24.765, 17.78)
  line L71 (26.035, 17.78) -> (26.67, 17.145)
  arc A128 (33.6191, 15.2759) -> (33.6909, 15.2041) centre (33.655, 15.24) ccw
  arc A129 (28.575, 15.1892) -> (28.575, 15.2908) centre (28.575, 15.24) ccw
  line L72 (34.29, 15.875) -> (33.655, 15.24)
  line L73 (32.385, 17.78) -> (33.655, 17.78)
  line L74 (24.765, 17.78) -> (26.035, 17.78)
  arc A130 (32.3491, 15.2041) -> (32.4209, 15.2759) centre (32.385, 15.24) ccw
  arc A131 (27.305, 15.2908) -> (27.305, 15.1892) centre (27.305, 15.24) ccw
  arc A132 (27.305, 17.8308) -> (27.305, 17.7292) centre (27.305, 17.78) ccw
  line L75 (29.845, 17.78) -> (29.21, 17.145)
  line L76 (24.13, 15.875) -> (23.495, 15.24)
  arc A133 (22.225, 17.8308) -> (22.225, 17.7292) centre (22.225, 17.78) ccw
  arc A134 (24.0941, 17.1091) -> (24.1659, 17.1809) centre (24.13, 17.145) ccw
  arc A135 (29.2459, 15.9109) -> (29.1741, 15.8391) centre (29.21, 15.875) ccw
  arc A136 (24.1659, 15.8391) -> (24.0941, 15.9109) centre (24.13, 15.875) ccw
  arc A137 (24.8009, 17.7441) -> (24.7291, 17.8159) centre (24.765, 17.78) ccw
  arc A138 (32.385, 17.8308) -> (32.385, 17.7292) centre (32.385, 17.78) ccw
  line L77 (33.655, 17.78) -> (34.29, 17.145)
  arc A139 (34.3259, 15.8391) -> (34.2541, 15.9109) centre (34.29, 15.875) ccw
  arc A140 (31.7859, 15.9109) -> (31.7141, 15.8391) centre (31.75, 15.875) ccw
  line L78 (32.385, 15.24) -> (31.75, 15.875)
  arc A141 (26.035, 17.7292) -> (26.035, 17.8308) centre (26.035, 17.78) ccw
  arc A142 (34.2541, 17.1091) -> (34.3259, 17.1809) centre (34.29, 17.145) ccw
  line L79 (31.115, 15.24) -> (29.845, 15.24)
  arc A143 (32.4209, 17.7441) -> (32.3491, 17.8159) centre (32.385, 17.78) ccw
  arc A144 (27.3409, 17.7441) -> (27.2691, 17.8159) centre (27.305, 17.78) ccw
  arc A145 (26.7059, 15.9109) -> (26.6341, 15.8391) centre (26.67, 15.875) ccw
  arc A146 (23.5309, 17.8159) -> (23.4591, 17.7441) centre (23.495, 17.78) ccw
  line L80 (28.575, 15.24) -> (27.305, 15.24)
  arc A147 (41.8741, 17.1091) -> (41.9459, 17.1809) centre (41.91, 17.145) ccw
  arc A148 (24.0941, 17.1809) -> (24.1659, 17.1091) centre (24.13, 17.145) ccw
  line L81 (27.305, 17.78) -> (28.575, 17.78)
  arc A149 (31.115, 15.1892) -> (31.115, 15.2908) centre (31.115, 15.24) ccw
  arc A150 (29.1741, 17.1091) -> (29.2459, 17.1809) centre (29.21, 17.145) ccw
  arc A151 (32.385, 15.2908) -> (32.385, 15.1892) centre (32.385, 15.24) ccw
  arc A152 (26.6341, 17.1809) -> (26.7059, 17.1091) centre (26.67, 17.145) ccw
  arc A153 (28.5391, 15.2759) -> (28.6109, 15.2041) centre (28.575, 15.24) ccw
  arc A154 (26.6341, 17.1091) -> (26.7059, 17.1809) centre (26.67, 17.145) ccw
  line L82 (23.495, 17.78) -> (24.13, 17.145)
  arc A155 (28.6109, 17.8159) -> (28.5391, 17.7441) centre (28.575, 17.78) ccw
  arc A156 (21.5541, 17.1809) -> (21.6259, 17.1091) centre (21.59, 17.145) ccw
  line L83 (28.575, 17.78) -> (29.21, 17.145)
  line L84 (29.21, 15.875) -> (28.575, 15.24)
  line L85 (29.21, 15.875) -> (29.845, 15.24)
  arc A157 (29.1741, 17.1809) -> (29.2459, 17.1091) centre (29.21, 17.145) ccw
  arc A158 (31.7859, 15.8391) -> (31.7141, 15.9109) centre (31.75, 15.875) ccw
  arc A159 (23.4591, 15.2759) -> (23.5309, 15.2041) centre (23.495, 15.24) ccw
  arc A160 (29.2459, 15.8391) -> (29.1741, 15.9109) centre (29.21, 15.875) ccw
  arc A161 (28.575, 17.7292) -> (28.575, 17.8308) centre (28.575, 17.78) ccw
  arc A162 (23.495, 17.7292) -> (23.495, 17.8308) centre (23.495, 17.78) ccw
  line L86 (22.225, 17.78) -> (23.495, 17.78)
  arc A163 (31.7141, 17.1809) -> (31.7859, 17.1091) centre (31.75, 17.145) ccw
  arc A164 (33.6909, 17.8159) -> (33.6191, 17.7441) centre (33.655, 17.78) ccw
  arc A165 (29.8091, 15.2041) -> (29.8809, 15.2759) centre (29.845, 15.24) ccw
  line L87 (33.655, 15.24) -> (32.385, 15.24)
  arc A166 (26.0709, 17.8159) -> (25.9991, 17.7441) centre (26.035, 17.78) ccw
  arc A167 (33.655, 15.1892) -> (33.655, 15.2908) centre (33.655, 15.24) ccw
  arc A168 (24.765, 17.8308) -> (24.765, 17.7292) centre (24.765, 17.78) ccw
  line L88 (27.305, 15.24) -> (26.67, 15.875)
  arc A169 (33.655, 17.7292) -> (33.655, 17.8308) centre (33.655, 17.78) ccw
  line L89 (26.035, 15.24) -> (24.765, 15.24)
  arc A170 (21.6259, 15.9109) -> (21.5541, 15.8391) centre (21.59, 15.875) ccw
  arc A171 (3.5433, 5.0673) -> (4.1317, 3.8643) centre (5.067, 5.0672) ccw
  arc A172 (40.005, 17.8308) -> (40.005, 17.7292) centre (40.005, 17.78) ccw
  arc A173 (6.5913, 5.0673) -> (5.9817, 6.2865) centre (5.0675, 5.0674) ccw
  arc A174 (3.0353, 5.0673) -> (3.7547, 3.5161) centre (5.0674, 5.0673) ccw
  arc A175 (6.3881, 7.3342) -> (6.3881, 7.2708) centre (6.3881, 7.3025) ccw
  arc A176 (26.7059, 15.8391) -> (26.6341, 15.9109) centre (26.67, 15.875) ccw
  arc A177 (4.0591, 6.8316) -> (3.0353, 5.0673) centre (5.0676, 5.0672) ccw
  arc A178 (41.8592, 15.875) -> (41.9608, 15.875) centre (41.91, 15.875) ccw
  arc A179 (7.1755, 7.2708) -> (7.1755, 7.3342) centre (7.1755, 7.3025) ccw
  arc A180 (6.3682, 3.5063) -> (7.0993, 5.0673) centre (5.0675, 5.0672) ccw
  arc A181 (41.275, 17.7292) -> (41.275, 17.8308) centre (41.275, 17.78) ccw
  arc A182 (21.5392, 15.875) -> (21.6408, 15.875) centre (21.59, 15.875) ccw
  line L90 (22.225, 17.78) -> (21.59, 17.145)
  arc A183 (9.098, 33.2692) -> (9.098, 33.3708) centre (9.098, 33.32) ccw
  arc A184 (1.9872, 33.32) -> (2.0888, 33.32) centre (2.038, 33.32) ccw
  line L91 (23.495, 15.24) -> (22.225, 15.24)
  line L92 (2.038, 45.42) -> (9.098, 45.42)
  arc A185 (24.7291, 15.2041) -> (24.8009, 15.2759) centre (24.765, 15.24) ccw
  arc A186 (41.275, 15.1892) -> (41.275, 15.2908) centre (41.275, 15.24) ccw
  arc A187 (26.035, 15.1892) -> (26.035, 15.2908) centre (26.035, 15.24) ccw
  arc A188 (25.9991, 15.2759) -> (26.0709, 15.2041) centre (26.035, 15.24) ccw
  arc A189 (21.6408, 17.145) -> (21.5392, 17.145) centre (21.59, 17.145) ccw
  line L93 (21.59, 15.875) -> (22.225, 15.24)
  arc A190 (41.3109, 17.8159) -> (41.2391, 17.7441) centre (41.275, 17.78) ccw
  line L94 (41.275, 15.24) -> (40.005, 15.24)
  line L95 (41.91, 15.875) -> (41.275, 15.24)
  arc A191 (39.9691, 15.2041) -> (40.0409, 15.2759) centre (40.005, 15.24) ccw
  arc A192 (23.495, 15.1892) -> (23.495, 15.2908) centre (23.495, 15.24) ccw
  line L96 (21.59, 17.145) -> (21.59, 15.875)
  arc A193 (24.765, 15.2908) -> (24.765, 15.1892) centre (24.765, 15.24) ccw
  line L97 (9.098, 33.32) -> (9.098, 45.42)
  arc A194 (22.225, 15.2908) -> (22.225, 15.1892) centre (22.225, 15.24) ccw
  arc A195 (41.2391, 15.2759) -> (41.3109, 15.2041) centre (41.275, 15.24) ccw
  arc A196 (39.3341, 17.1809) -> (39.4059, 17.1091) centre (39.37, 17.145) ccw
  arc A197 (2.0888, 45.42) -> (1.9872, 45.42) centre (2.038, 45.42) ccw
  line L98 (24.765, 15.24) -> (24.13, 15.875)
  arc A198 (9.0472, 33.32) -> (9.1488, 33.32) centre (9.098, 33.32) ccw
  arc A199 (2.038, 33.3708) -> (2.038, 33.2692) centre (2.038, 33.32) ccw
  arc A200 (9.098, 45.3692) -> (9.098, 45.4708) centre (9.098, 45.42) ccw
  arc A201 (41.9608, 17.145) -> (41.8592, 17.145) centre (41.91, 17.145) ccw
  arc A202 (40.0409, 17.7441) -> (39.9691, 17.8159) centre (40.005, 17.78) ccw
  line L99 (2.038, 45.42) -> (2.038, 33.32)
  line L100 (40.005, 17.78) -> (39.37, 17.145)
  arc A203 (40.005, 15.2908) -> (40.005, 15.1892) centre (40.005, 15.24) ccw
  arc A204 (39.4059, 15.9109) -> (39.3341, 15.8391) centre (39.37, 15.875) ccw
  line L101 (40.005, 17.78) -> (41.275, 17.78)
  arc A205 (2.038, 45.4708) -> (2.038, 45.3692) centre (2.038, 45.42) ccw
  line L102 (6.7945, 7.6581) -> (6.7945, 6.9215)
  line L103 (41.275, 17.78) -> (41.91, 17.145)
  arc A206 (22.1891, 15.2041) -> (22.2609, 15.2759) centre (22.225, 15.24) ccw
  line L104 (41.91, 17.145) -> (41.91, 15.875)
  line L105 (9.098, 33.32) -> (2.038, 33.32)
  arc A207 (6.7628, 6.9215) -> (6.8262, 6.9215) centre (6.7945, 6.9215) ccw
  arc A208 (6.8262, 7.6581) -> (6.7628, 7.6581) centre (6.7945, 7.6581) ccw
  line L106 (26.67, 15.875) -> (26.035, 15.24)
  arc A209 (41.9459, 15.8391) -> (41.8741, 15.9109) centre (41.91, 15.875) ccw
  arc A210 (9.1488, 45.42) -> (9.0472, 45.42) centre (9.098, 45.42) ccw
  arc A211 (7.0993, 5.0673) -> (6.0235, 6.8602) centre (5.0674, 5.0673) ccw
  line L107 (39.37, 15.875) -> (40.005, 15.24)
  arc A212 (22.2609, 17.7441) -> (22.1891, 17.8159) centre (22.225, 17.78) ccw
  line L108 (6.3881, 7.3025) -> (7.1755, 7.3025)
  arc A213 (24.1659, 15.9109) -> (24.0941, 15.8391) centre (24.13, 15.875) ccw
  arc A214 (74.676, 13.5509) -> (74.676, 13.6271) centre (74.676, 13.589) ccw
  line L109 (80.772, 11.557) -> (80.772, 13.335)
  arc A215 (75.1571, 13.4351) -> (75.2109, 13.4889) centre (75.184, 13.462) ccw
  line L110 (80.01, 11.43) -> (80.137, 11.303)
  arc A216 (75.184, 13.5001) -> (75.184, 13.4239) centre (75.184, 13.462) ccw
  arc A217 (74.676, 11.2649) -> (74.676, 11.3411) centre (74.676, 11.303) ccw
  arc A218 (74.676, 13.589) -> (74.422, 13.335) centre (74.676, 13.335) ccw
  line L111 (74.676, 13.589) -> (75.057, 13.589)
  line L112 (81.6356, 12.1412) -> (81.6356, 12.7508)
  arc A219 (80.518, 11.2649) -> (80.518, 11.3411) centre (80.518, 11.303) ccw
  arc A220 (14.8558, 3.8399) -> (15.494, 5.08) centre (13.97, 5.0801) ccw
  arc A221 (80.518, 13.6271) -> (80.518, 13.5509) centre (80.518, 13.589) ccw
  arc A222 (13.0344, 6.283) -> (12.446, 5.08) centre (13.9697, 5.0801) ccw
  arc A223 (15.2908, 7.3469) -> (15.2908, 7.2835) centre (15.2908, 7.3152) ccw
  line L113 (15.6972, 7.6708) -> (15.6972, 6.9342)
  arc A224 (74.3839, 13.335) -> (74.4601, 13.335) centre (74.422, 13.335) ccw
  arc A225 (80.518, 11.3411) -> (80.518, 11.2649) centre (80.518, 11.303) ccw
  arc A226 (11.938, 5.08) -> (12.6574, 3.5288) centre (13.9701, 5.08) ccw
  arc A227 (15.6654, 6.9342) -> (15.729, 6.9342) centre (15.6972, 6.9342) ccw
  arc A228 (5.9531, 3.8272) -> (6.5913, 5.0673) centre (5.0673, 5.0674) ccw
  arc A229 (15.729, 7.6708) -> (15.6654, 7.6708) centre (15.6972, 7.6708) ccw
  arc A230 (80.7339, 11.557) -> (80.8101, 11.557) centre (80.772, 11.557) ccw
  arc A231 (75.0301, 11.3299) -> (75.0839, 11.2761) centre (75.057, 11.303) ccw
  arc A232 (15.494, 5.08) -> (14.8844, 6.2992) centre (13.9702, 5.0801) ccw
  arc A233 (12.9618, 6.8443) -> (11.938, 5.08) centre (13.9703, 5.0799) ccw
  arc A234 (80.01, 11.3919) -> (80.01, 11.4681) centre (80.01, 11.43) ccw
  arc A235 (74.422, 11.557) -> (74.676, 11.303) centre (74.676, 11.557) ccw
  line L114 (80.772, 12.1412) -> (81.6356, 12.1412)
  line L115 (81.6356, 12.7508) -> (80.772, 12.7508)
  line L116 (80.518, 11.303) -> (80.137, 11.303)
  arc A236 (75.057, 11.2649) -> (75.057, 11.3411) centre (75.057, 11.303) ccw
  arc A237 (74.676, 11.3411) -> (74.676, 11.2649) centre (74.676, 11.303) ccw
  arc A238 (12.446, 5.08) -> (13.0344, 3.877) centre (13.9697, 5.0799) ccw
  line L117 (15.2908, 7.3152) -> (16.0782, 7.3152)
  arc A239 (80.518, 11.303) -> (80.772, 11.557) centre (80.518, 11.557) ccw
  arc A240 (74.3839, 11.557) -> (74.4601, 11.557) centre (74.422, 11.557) ccw
  arc A241 (80.1639, 13.5621) -> (80.1101, 13.6159) centre (80.137, 13.589) ccw
  arc A242 (4.1317, 6.2703) -> (3.5433, 5.0673) centre (5.067, 5.0674) ccw
  arc A243 (80.1101, 11.2761) -> (80.1639, 11.3299) centre (80.137, 11.303) ccw
  arc A244 (80.772, 13.335) -> (80.518, 13.589) centre (80.518, 13.335) ccw
  arc A245 (80.137, 13.6271) -> (80.137, 13.5509) centre (80.137, 13.589) ccw
  arc A246 (16.002, 5.08) -> (14.9262, 6.8729) centre (13.9701, 5.08) ccw
  arc A247 (15.2709, 3.519) -> (16.002, 5.08) centre (13.9702, 5.0799) ccw
  line L118 (73.5584, 12.7508) -> (73.5584, 12.1412)
  line L119 (80.01, 11.43) -> (75.184, 11.43)
  line L120 (75.184, 13.462) -> (75.057, 13.589)
  line L121 (74.676, 11.303) -> (75.057, 11.303)
  arc A248 (74.676, 13.6271) -> (74.676, 13.5509) centre (74.676, 13.589) ccw
  arc A249 (79.9831, 13.4889) -> (80.0369, 13.4351) centre (80.01, 13.462) ccw
  arc A250 (74.4601, 11.557) -> (74.3839, 11.557) centre (74.422, 11.557) ccw
  arc A251 (75.0839, 13.6159) -> (75.0301, 13.5621) centre (75.057, 13.589) ccw
  line L122 (80.772, 12.7508) -> (80.772, 12.1412)
  arc A252 (16.0782, 7.2835) -> (16.0782, 7.3469) centre (16.0782, 7.3152) ccw
  arc A253 (75.2109, 11.4031) -> (75.1571, 11.4569) centre (75.184, 11.43) ccw
  arc A254 (80.0369, 11.4569) -> (79.9831, 11.4031) centre (80.01, 11.43) ccw
  arc A255 (80.7339, 13.335) -> (80.8101, 13.335) centre (80.772, 13.335) ccw
  line L123 (74.422, 12.7508) -> (73.5584, 12.7508)
  arc A256 (80.8101, 11.557) -> (80.7339, 11.557) centre (80.772, 11.557) ccw
  arc A257 (80.137, 11.3411) -> (80.137, 11.2649) centre (80.137, 11.303) ccw
  arc A258 (75.184, 11.4681) -> (75.184, 11.3919) centre (75.184, 11.43) ccw
  line L124 (75.184, 11.43) -> (75.057, 11.303)
  line L125 (80.01, 13.462) -> (80.137, 13.589)
  line L126 (80.01, 13.462) -> (75.184, 13.462)
  arc A259 (75.057, 13.5509) -> (75.057, 13.6271) centre (75.057, 13.589) ccw
  line L127 (73.5584, 12.1412) -> (74.422, 12.1412)
  arc A260 (13.1064, 10.3124) -> (13.1064, 10.2362) centre (13.1064, 10.2743) ccw
  arc A261 (7.2644, 12.5603) -> (7.0104, 12.3063) centre (7.2644, 12.3063) ccw
  arc A262 (7.6185, 10.3012) -> (7.6723, 10.2474) centre (7.6454, 10.2743) ccw
  line L128 (14.224, 11.1125) -> (14.224, 11.7221)
  line L129 (74.422, 12.1412) -> (74.422, 12.7508)
  arc A263 (7.7724, 10.4394) -> (7.7724, 10.3632) centre (7.7724, 10.4013) ccw
  arc A264 (12.7523, 12.5334) -> (12.6985, 12.5872) centre (12.7254, 12.5603) ccw
  arc A265 (13.1064, 10.2362) -> (13.1064, 10.3124) centre (13.1064, 10.2743) ccw
  line L130 (12.5984, 10.4013) -> (12.7254, 10.2743)
  arc A266 (13.1064, 12.5984) -> (13.1064, 12.5222) centre (13.1064, 12.5603) ccw
  line L131 (80.518, 13.589) -> (80.137, 13.589)
  arc A267 (13.3223, 12.3063) -> (13.3985, 12.3063) centre (13.3604, 12.3063) ccw
  arc A268 (12.5984, 10.3632) -> (12.5984, 10.4394) centre (12.5984, 10.4013) ccw
  arc A269 (12.5715, 12.4602) -> (12.6253, 12.4064) centre (12.5984, 12.4333) ccw
  line L132 (7.0104, 12.3063) -> (7.0104, 10.5283)
  arc A270 (12.6985, 10.2474) -> (12.7523, 10.3012) centre (12.7254, 10.2743) ccw
  line L133 (7.7724, 10.4013) -> (12.5984, 10.4013)
  arc A271 (7.7455, 12.4064) -> (7.7993, 12.4602) centre (7.7724, 12.4333) ccw
  arc A272 (12.7254, 12.5984) -> (12.7254, 12.5222) centre (12.7254, 12.5603) ccw
  arc A273 (7.2644, 12.5984) -> (7.2644, 12.5222) centre (7.2644, 12.5603) ccw
  line L134 (13.3604, 12.3063) -> (13.3604, 10.5283)
  line L135 (7.7724, 10.4013) -> (7.6454, 10.2743)
  arc A274 (12.7254, 10.3124) -> (12.7254, 10.2362) centre (12.7254, 10.2743) ccw
  arc A275 (13.3223, 10.5283) -> (13.3985, 10.5283) centre (13.3604, 10.5283) ccw
  arc A276 (74.4601, 13.335) -> (74.3839, 13.335) centre (74.422, 13.335) ccw
  line L136 (14.224, 11.7221) -> (13.3604, 11.7221)
  arc A277 (7.2644, 10.3124) -> (7.2644, 10.2362) centre (7.2644, 10.2743) ccw
  arc A278 (13.1064, 10.2743) -> (13.3604, 10.5283) centre (13.1064, 10.5283) ccw
  arc A279 (7.7993, 10.3744) -> (7.7455, 10.4282) centre (7.7724, 10.4013) ccw
  arc A280 (7.0485, 10.5283) -> (6.9723, 10.5283) centre (7.0104, 10.5283) ccw
  arc A281 (7.2644, 12.5222) -> (7.2644, 12.5984) centre (7.2644, 12.5603) ccw
  arc A282 (13.3604, 12.3063) -> (13.1064, 12.5603) centre (13.1064, 12.3063) ccw
  line L137 (74.422, 11.557) -> (74.422, 13.335)
  arc A283 (7.6454, 10.2362) -> (7.6454, 10.3124) centre (7.6454, 10.2743) ccw
  arc A284 (7.6723, 12.5872) -> (7.6185, 12.5334) centre (7.6454, 12.5603) ccw
  line L138 (7.7724, 12.4333) -> (7.6454, 12.5603)
  line L139 (13.1064, 12.5603) -> (12.7254, 12.5603)
  arc A285 (7.6454, 12.5222) -> (7.6454, 12.5984) centre (7.6454, 12.5603) ccw
  line L140 (13.3604, 11.1125) -> (14.224, 11.1125)